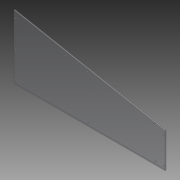
# Autodesk Inventor part: Hopper Front
Saved by Autodesk Inventor 2014 SP1 (Build 180222100, 222)
## iProperties
Created: 2013-12-16
Part Number: Hopper Front
Material: Polycarbonate, Clear
Document SubType Name: Modeling
Designer: Moses
Density: 1.2 g/cm^3
Appearance: Polycarbonate - Clear
Mass: 271.411 g
Surface Area: 1469.16 cm^2
Volume: 226.176 cm^3
Author: Moses
Autodesk Inventor part; units mm, degrees
ref_plane "YZ Plane" through (0, 0, 0) normal (1, 0, 0) x (0, 1, 0)
ref_plane "XZ Plane" through (0, 0, 0) normal (0, 1, 0) x (-1, 0, 0)
ref_plane "XY Plane" through (0, 0, 0) normal (0, 0, 1) x (1, 0, 0)
sketch "Sketch1" plane through (0, 0, 0) normal (0, 0, 1) x (1, 0, 0)
  line L0 (467.8685, 107.8942) -> (0, 196.85)
  line L1 (0, 0) -> (467.8685, 0)
  line L2 (0, 196.85) -> (0, 0)
  line L3 (467.8685, 107.8942) -> (467.8685, 0)
  line L4 (467.8685, 0) -> (468.4718, 0)
  line L5 (468.4718, 0) -> (468.4718, 107.7795)
  line L6 (468.4718, 107.7795) -> (467.8685, 107.8942)
  circle A0 centre (295.5085, 133.0828) radius 1.5875
  circle A1 centre (432.753, 107.0054) radius 1.5875
  circle A2 centre (364.1308, 120.0441) radius 1.5875
  circle A3 centre (226.8862, 146.1214) radius 1.5875
  line L7 (443.6664, 113.4153) -> (440.703, 97.8194) construction
  line L8 (443.6664, 113.4153) -> (219.0844, 156.0873) construction
  line L9 (216.1211, 140.4914) -> (219.0844, 156.0873) construction
  line L10 (440.703, 97.8194) -> (216.1211, 140.4914) construction
  circle A4 centre (230.3468, 7.5406) radius 1.5875
  circle A5 centre (436.7218, 7.5406) radius 1.5875
  circle A6 centre (23.9718, 7.5406) radius 1.5875
  line L11 (446.2468, 15.0813) -> (446.2468, -0.7937) construction
  line L12 (446.2468, 15.0813) -> (14.4468, 15.0813) construction
  line L13 (14.4468, -0.7937) -> (14.4468, 15.0813) construction
  line L14 (446.2468, -0.7937) -> (14.4468, -0.7937) construction
  circle A7 centre (4.3656, 95.25) radius 1.5875
  circle A8 centre (4.3656, 177.8) radius 1.5875
  circle A9 centre (4.3656, 12.7) radius 1.5875
  line L15 (-3.9687, 190.5) -> (11.9063, 190.5) construction
  line L16 (-3.9687, 190.5) -> (-3.9687, 0) construction
  line L17 (11.9063, 0) -> (-3.9687, 0) construction
  line L18 (11.9063, 190.5) -> (11.9063, 0) construction
  circle A10 centre (464.1061, 8.7313) radius 1.5875
  circle A11 centre (464.1061, 91.2812) radius 1.5875
  line L19 (456.5655, -0.7937) -> (471.6468, -0.7937) construction
  line L20 (456.5655, -0.7937) -> (456.5655, 100.8062) construction
  line L21 (471.6468, 100.8062) -> (456.5655, 100.8062) construction
  line L22 (471.6468, -0.7937) -> (471.6468, 100.8062) construction
  circle A12 centre (71.5968, 99.6156) radius 1.5875
  line L23 (81.1218, 107.95) -> (81.1218, 92.075) construction
  line L24 (81.1218, 107.95) -> (62.0718, 107.95) construction
  line L25 (62.0718, 92.075) -> (62.0718, 107.95) construction
  line L26 (81.1218, 92.075) -> (62.0718, 92.075) construction
  circle A13 centre (243.0468, 99.6156) radius 1.5875
  line L27 (252.5718, 107.95) -> (252.5718, 92.075) construction
  line L28 (252.5718, 107.95) -> (233.5218, 107.95) construction
  line L29 (233.5218, 92.075) -> (233.5218, 107.95) construction
  line L30 (252.5718, 92.075) -> (233.5218, 92.075) construction
  circle A14 centre (158.75, 154.8401) radius 1.5875
  line L31 (146.05, 145.3151) -> (146.05, 158.0151) construction
  line L32 (146.05, 145.3151) -> (171.45, 145.3151) construction
  line L33 (171.45, 158.0151) -> (171.45, 145.3151) construction
  line L34 (146.05, 158.0151) -> (171.45, 158.0151) construction
extrude "Extrusion1" add sketch "Sketch1" along normal blind 3.175
body "Solid1"
